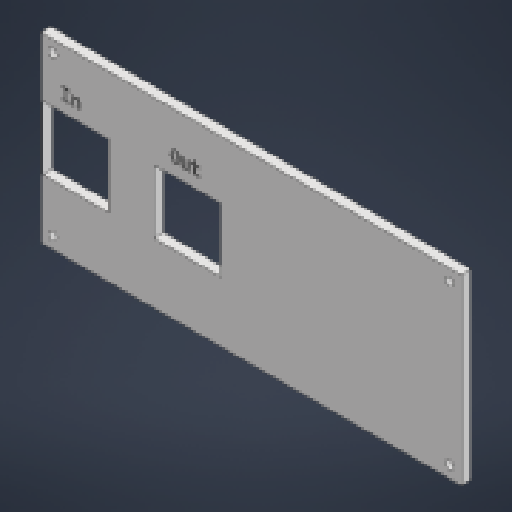
# Autodesk Inventor part: backplate_lvl202x01
Saved by Autodesk Inventor 2024 (Build 280153000, 153)
## iProperties
Created: 2026-05-08
Part Number: backplate_lvl202x01
Material: Generic
Document SubType Name: Modeling
Designer: schar
Density: 1 g/cm^3
Appearance: Default
Author: schar
Autodesk Inventor part; units mm, degrees
ref_plane "YZ Plane" through (0, 0, 0) normal (1, 0, 0) x (0, 1, 0)
ref_plane "XZ Plane" through (0, 0, 0) normal (0, 1, 0) x (-1, 0, 0)
ref_plane "XY Plane" through (0, 0, 0) normal (0, 0, 1) x (1, 0, 0)
sketch "Sketch1" plane through (0, 0, 0) normal (0, 0, 1) x (1, 0, 0)
  line L0 (-112.7024, 42.5741) -> (-128.5024, 42.5741) projected
  line L1 (-112.2524, 27.0241) -> (-112.2524, 42.1241) projected
  line L2 (-100.8524, 42.2341) -> (-100.8524, 27.1341) projected
  line L3 (-84.6024, 42.6841) -> (-100.4024, 42.6841) projected
  line L4 (-84.1524, 27.1341) -> (-84.1524, 32.1691) projected
  line L5 (-100.4024, 26.6841) -> (-84.6024, 26.6841) projected
  line L6 (-128.5024, 26.5741) -> (-112.7024, 26.5741) projected
  line L7 (-128.9524, 32.0591) -> (-128.9524, 27.0241) projected
  circle A0 centre (-126.4024, 54.4141) radius 1.1 projected
  circle A1 centre (-126.4024, 14.4141) radius 1.1 projected
  line L8 (-129.6024, 11.2141) -> (-129.6024, 57.6141) projected
  line L9 (-23.2024, 11.2141) -> (-129.6024, 11.2141) projected
  line L10 (-23.2024, 57.6141) -> (-23.2024, 11.2141) projected
  line L11 (-129.6024, 57.6141) -> (-23.2024, 57.6141) projected
  line L12 (-112.7024, 26.5741) -> (-108.9398, 26.5741)
  line L13 (-112.2524, 27.0241) -> (-112.2524, 26.5741)
  line L14 (-128.5024, 42.5741) -> (-131.0464, 42.5741)
  line L15 (-128.9524, 32.0591) -> (-128.9524, 42.5741)
  line L16 (-128.9524, 42.5741) -> (-112.2524, 42.5741)
  line L17 (-112.2524, 42.5741) -> (-112.2524, 26.5741)
  line L18 (-112.2524, 26.5741) -> (-128.9524, 26.5741)
  line L19 (-128.9524, 26.5741) -> (-128.9524, 42.5741)
  line L20 (-100.4024, 26.6841) -> (-102.0076, 26.6841)
  line L21 (-100.8524, 27.1341) -> (-100.8524, 26.6841)
  line L22 (-84.1524, 32.1691) -> (-84.1524, 43.4133)
  line L23 (-84.6024, 42.6841) -> (-84.1524, 42.6841)
  line L24 (-84.1524, 42.6841) -> (-100.8524, 42.6841)
  line L25 (-100.8524, 42.6841) -> (-100.8524, 26.6841)
  line L26 (-100.8524, 26.6841) -> (-84.1524, 26.6841)
  line L27 (-84.1524, 26.6841) -> (-84.1524, 42.6841)
  line L28 (-23.2024, 57.6141) -> (-26.4024, 57.6141)
  line L29 (-26.4024, 57.6141) -> (-26.4024, 54.4141)
  circle A2 centre (-26.4024, 54.4141) radius 1.1
  line L30 (-23.2024, 11.2141) -> (-21.0735, 11.2141)
  line L31 (-21.0735, 11.2141) -> (-21.0735, 8.0141)
  circle A3 centre (-21.0735, 8.0141) radius 1.1
  line L32 (-23.4024, 57.4141) -> (-23.4024, 11.4141)
  line L33 (-23.4024, 11.4141) -> (-129.4024, 11.4141)
  line L34 (-129.4024, 11.4141) -> (-129.4024, 57.4141)
  line L35 (-129.4024, 57.4141) -> (-23.4024, 57.4141)
  point P0 (0, 0)
  point P1 (-128.9524, 32.0583)
  point P2 (-46.5566, -2.8057)
  point P3 (-1.7566, -2.6957)
  dimension "d0" = 3.2
  dimension "d1" = 3.2
  dimension "d2" = 2.2
  dimension "d3" = 3.2
  dimension "d4" = 2.2
  dimension "d7" = 0.2
  constraints: 48 end point, 6 perpendicular, 6 point on line, 4 horizontal, 4 parallel, 3 collinear, 3 vertical, 2 centre point, 2 coincident, 3 other
  measures "d0" distance of L10.start L28.end
  measures "d1" distance of L28.end L29.end
  measures "d2" diameter of A2
  measures "d3" distance of L30.end L31.end
  measures "d4" diameter of A3
  measures "d7" distance between parallel lines of L11 L35
extrude "Extrusion1" add sketch "Sketch1" against normal blind 2.5 contours L34 L35 L32 L33
sketch "Sketch2" plane through (0, 0, 0) normal (0, 0, 1) x (1, 0, 0)
  circle A0 centre (-26.4024, 14.4141) radius 1.1 projected
  point P0 (0, 0)
extrude "Extrusion2" cut sketch "Sketch2" against normal blind 2.5
sketch "Sketch3" plane through (0, 0, 0) normal (0, 0, 1) x (1, 0, 0)
  line L0 (-124.4974, 48.3763) -> (-113.1693, 48.3763) construction
  line L1 (-113.1693, 48.3763) -> (-113.1693, 42.6829) construction
  line L2 (-113.1693, 42.6829) -> (-124.4974, 42.6829) construction
  line L3 (-124.4974, 42.6829) -> (-124.4974, 48.3763) construction
  line L4 (-96.8522, 48.7284) -> (-79.8895, 48.7284) construction
  line L5 (-79.8895, 48.7284) -> (-79.8895, 44.5024) construction
  line L6 (-79.8895, 44.5024) -> (-96.8522, 44.5024) construction
  line L7 (-96.8522, 44.5024) -> (-96.8522, 48.7284) construction
  line L8 (-123.3932, 48.0264) -> (-124.0956, 48.0264)
  line L9 (-124.0956, 48.0264) -> (-124.0956, 48.3763)
  line L10 (-124.0956, 48.3763) -> (-122.27, 48.3763)
  line L11 (-122.27, 48.3763) -> (-122.27, 48.0264)
  line L12 (-122.27, 48.0264) -> (-122.9724, 48.0264)
  line L13 (-122.9724, 48.0264) -> (-122.9724, 45.6816)
  line L14 (-122.9724, 45.6816) -> (-122.27, 45.6816)
  line L15 (-122.27, 45.6816) -> (-122.27, 45.3263)
  line L16 (-122.27, 45.3263) -> (-124.0956, 45.3263)
  line L17 (-124.0956, 45.3263) -> (-124.0956, 45.6816)
  line L18 (-124.0956, 45.6816) -> (-123.3932, 45.6816)
  line L19 (-123.3932, 45.6816) -> (-123.3932, 48.0264)
  line L20 (-121.4938, 47.6684) -> (-121.1303, 47.6684)
  line L21 (-121.1303, 47.6684) -> (-121.1139, 47.2913)
  spline S0 degree 2 poles (-121.1139, 47.2913) (-121.0128, 47.4115) (-120.8215, 47.5728) (-120.6357, 47.6712) (-120.4444, 47.7122) (-120.3405, 47.7122) knots 0 0 0 1 2 3 4 4 4
  spline S1 degree 2 poles (-120.3405, 47.7122) (-119.9798, 47.7122) (-119.6081, 47.2858) (-119.6081, 46.8567) knots 0 0 0 1 2 2 2
  line L22 (-119.6081, 46.8567) -> (-119.6081, 45.3263)
  line L23 (-119.6081, 45.3263) -> (-120.0153, 45.3263)
  line L24 (-120.0153, 45.3263) -> (-120.0153, 46.8239)
  spline S2 degree 2 poles (-120.0153, 46.8239) (-120.0153, 47.0972) (-120.2203, 47.3623) (-120.4225, 47.3623) knots 0 0 0 1 2 2 2
  spline S3 degree 2 poles (-120.4225, 47.3623) (-120.499, 47.3623) (-120.6411, 47.3186) (-120.7942, 47.2093) (-120.9746, 47.0207) (-121.0866, 46.8813) knots 0 0 0 1 2 3 4 4 4
  line L25 (-121.0866, 46.8813) -> (-121.0866, 45.3263)
  line L26 (-121.0866, 45.3263) -> (-121.4938, 45.3263)
  line L27 (-121.4938, 45.3263) -> (-121.4938, 47.6684)
  spline S4 degree 2 poles (-94.3515, 47.1816) (-94.3515, 46.7689) (-94.5456, 46.1731) (-94.8735, 45.7823) (-95.3163, 45.5937) (-95.5595, 45.5937) knots 0 0 0 1 2 3 4 4 4
  spline S5 degree 2 poles (-95.5595, 45.5937) (-95.8547, 45.5937) (-96.2919, 45.8069) (-96.5789, 46.2086) (-96.7183, 46.7853) (-96.7183, 47.146) knots 0 0 0 1 2 3 4 4 4
  spline S6 degree 2 poles (-96.7183, 47.146) (-96.7183, 47.5533) (-96.527, 48.149) (-96.199, 48.5399) (-95.759, 48.7284) (-95.513, 48.7284) knots 0 0 0 1 2 3 4 4 4
  spline S7 degree 2 poles (-95.513, 48.7284) (-95.2206, 48.7284) (-94.7833, 48.5125) (-94.4936, 48.1135) (-94.3515, 47.5396) (-94.3515, 47.1816) knots 0 0 0 1 2 3 4 4 4
  spline S8 degree 2 poles (-94.7669, 47.1515) (-94.7669, 47.4193) (-94.8517, 47.8648) (-95.0375, 48.1873) (-95.3299, 48.365) (-95.5376, 48.365) knots 0 0 0 1 2 3 4 4 4
  spline S9 degree 2 poles (-95.5376, 48.365) (-95.7371, 48.365) (-96.0268, 48.1764) (-96.2127, 47.8512) (-96.3029, 47.4139) (-96.3029, 47.1679) knots 0 0 0 1 2 3 4 4 4
  spline S10 degree 2 poles (-96.3029, 47.1679) (-96.3029, 46.8973) (-96.2181, 46.4519) (-96.0323, 46.1321) (-95.7426, 45.9545) (-95.5376, 45.9545) knots 0 0 0 1 2 3 4 4 4
  spline S11 degree 2 poles (-95.5376, 45.9545) (-95.3381, 45.9545) (-95.0457, 46.143) (-94.8571, 46.4683) (-94.7669, 46.9028) (-94.7669, 47.1515) knots 0 0 0 1 2 3 4 4 4
  line L28 (-91.9629, 45.6347) -> (-92.3291, 45.6347)
  line L29 (-92.3291, 45.6347) -> (-92.3428, 46.0119)
  spline S12 degree 2 poles (-92.3428, 46.0119) (-92.4466, 45.8916) (-92.6352, 45.7304) (-92.8238, 45.632) (-93.0124, 45.5937) (-93.1162, 45.5937) knots 0 0 0 1 2 3 4 4 4
  spline S13 degree 2 poles (-93.1162, 45.5937) (-93.4797, 45.5937) (-93.8487, 46.0173) (-93.8487, 46.4464) knots 0 0 0 1 2 2 2
  line L30 (-93.8487, 46.4464) -> (-93.8487, 47.9769)
  line L31 (-93.8487, 47.9769) -> (-93.4414, 47.9769)
  line L32 (-93.4414, 47.9769) -> (-93.4414, 46.4792)
  spline S14 degree 2 poles (-93.4414, 46.4792) (-93.4414, 45.9408) (-93.0342, 45.9408) knots 0 0 0 1 1 1
  spline S15 degree 2 poles (-93.0342, 45.9408) (-92.9604, 45.9408) (-92.8183, 45.9845) (-92.6625, 46.0938) (-92.4822, 46.2824) (-92.3701, 46.4245) knots 0 0 0 1 2 3 4 4 4
  line L33 (-92.3701, 46.4245) -> (-92.3701, 47.9769)
  line L34 (-92.3701, 47.9769) -> (-91.9629, 47.9769)
  line L35 (-91.9629, 47.9769) -> (-91.9629, 45.6347)
  spline S16 degree 2 poles (-89.3311, 45.6675) (-89.4677, 45.632) (-89.7629, 45.6019) (-89.9159, 45.6019) knots 0 0 0 1 2 2 2
  spline S17 degree 2 poles (-89.9159, 45.6019) (-90.3559, 45.6019) (-90.7905, 46.0009) (-90.7905, 46.4136) knots 0 0 0 1 2 2 2
  line L36 (-90.7905, 46.4136) -> (-90.7905, 47.6352)
  line L37 (-90.7905, 47.6352) -> (-91.4464, 47.6352)
  line L38 (-91.4464, 47.6352) -> (-91.4464, 47.9769)
  line L39 (-91.4464, 47.9769) -> (-90.7905, 47.9769)
  line L40 (-90.7905, 47.9769) -> (-90.7905, 48.6219)
  line L41 (-90.7905, 48.6219) -> (-90.3832, 48.7257)
  line L42 (-90.3832, 48.7257) -> (-90.3832, 47.9769)
  line L43 (-90.3832, 47.9769) -> (-89.3311, 47.9769)
  line L44 (-89.3311, 47.9769) -> (-89.3311, 47.6352)
  line L45 (-89.3311, 47.6352) -> (-90.3832, 47.6352)
  line L46 (-90.3832, 47.6352) -> (-90.3832, 46.4464)
  spline S18 degree 2 poles (-90.3832, 46.4464) (-90.3832, 46.195) (-90.1154, 45.9463) (-89.8531, 45.9463) knots 0 0 0 1 2 2 2
  spline S19 degree 2 poles (-89.8531, 45.9463) (-89.741, 45.9463) (-89.4759, 45.9818) (-89.3311, 46.0173) knots 0 0 0 1 2 2 2
  line L47 (-89.3311, 46.0173) -> (-89.3311, 45.6675)
  point P0 (0, 0)
  constraints: 4 other
extrude "Extrusion3" cut sketch "Sketch3" against normal blind 0.2
body "Solid1"
